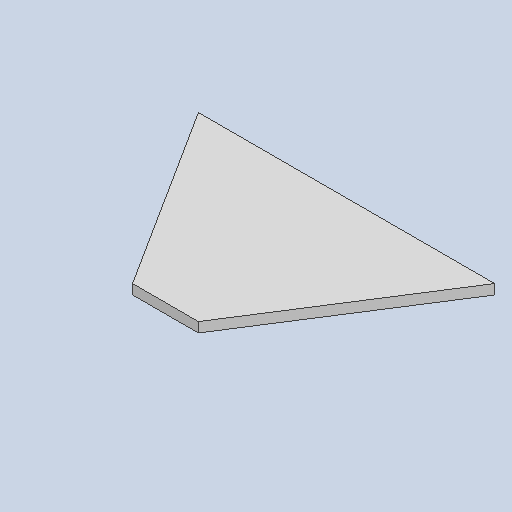
# Autodesk Inventor part: blacha_dolna_pre
Saved by Autodesk Inventor 2023 (Build 270158000, 158)
## iProperties
Created: 2024-06-27
Part Number: blacha_dolna_pre
Material: Ogólny
Document SubType Name: Modeling
Designer: kamil
Density: 1 g/cm^3
Appearance: Domyślna
Author: kamil
Autodesk Inventor part; units mm, degrees
ref_plane "YZ Plane" through (0, 0, 0) normal (1, 0, 0) x (0, 1, 0)
ref_plane "XZ Plane" through (0, 0, 0) normal (0, 1, 0) x (-1, 0, 0)
ref_plane "XY Plane" through (0, 0, 0) normal (0, 0, 1) x (1, 0, 0)
sketch "Szkic1" plane through (0, 0, 0) normal (0, 1, 0) x (-1, 0, 0)
  line L0 (3.5174, 9.2032) -> (-16.4826, 9.2032)
  line L1 (-16.4826, 9.2032) -> (-16.4826, -45.7968)
  line L2 (-16.4826, -45.7968) -> (3.5174, -45.7968)
  line L3 (3.5174, -45.7968) -> (3.5174, 9.2032)
  line L4 (3.5174, -45.7968) -> (38.5174, -45.7968)
  line L5 (-16.4826, -45.7968) -> (-51.4826, -45.7968)
  line L6 (-51.4826, -45.7968) -> (-16.4826, 9.2032)
  line L7 (3.5174, 9.2032) -> (38.5174, -45.7968)
  point P0 (0, 0)
  dimension "d0" = 20
  dimension "d1" = 55
  dimension "d2" = 35
  dimension "d3" = 35
  constraints: 16 end point, 3 horizontal, 2 parallel, 1 perpendicular
  measures "d0" distance of L2.end L1.end
  measures "d1" distance of L1.end L0.end
  measures "d2" distance of L2.end L4.end
  measures "d3" distance of L1.end L5.end
extrude "Wyciągnięcie proste1" add sketch "Szkic1" along normal blind 3
